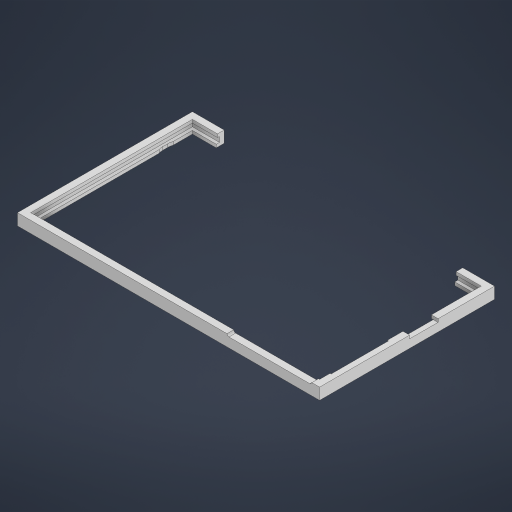
# Autodesk Inventor part: pcb_guard
Saved by Autodesk Inventor 2024 (Build 280153000, 153)
## iProperties
Created: 2024-03-10
Part Number: pcb_guard
Material: Všeobecné
Document SubType Name: Modeling
Designer: Simak
Density: 1 g/cm^3
Appearance: Výchozí
Author: Simak
Autodesk Inventor part; units mm, degrees
ref_plane "YZ Plane" through (0, 0, 0) normal (1, 0, 0) x (0, 1, 0)
ref_plane "XZ Plane" through (0, 0, 0) normal (0, 1, 0) x (-1, 0, 0)
ref_plane "XY Plane" through (0, 0, 0) normal (0, 0, 1) x (1, 0, 0)
sketch "Náčrt1" plane through (0, 0, 0) normal (0, 1, 0) x (-1, 0, 0)
  line L0 (47.5, -27.5) -> (-47.5, -27.5) construction
  line L1 (-47.5, -27.5) -> (-47.5, 27.5) construction
  line L2 (-47.5, 27.5) -> (47.5, 27.5) construction
  line L3 (47.5, 27.5) -> (47.5, -27.5) construction
  line L4 (47.5, -27.5) -> (0, 0) construction
  line L5 (0, 0) -> (-47.5, -27.5) construction
  line L6 (0, 0) -> (-47.5, 27.5) construction
  line L7 (-46, -26) -> (46, -26)
  line L8 (46, -26) -> (46, 26)
  line L9 (46, 26) -> (-46, 26)
  line L10 (-46, 26) -> (-46, -26)
  circle A0 centre (41, -16) radius 4.25
  circle A1 centre (41, -17.5) radius 4.25
  line L11 (45.25, -17.5) -> (45.25, -16)
  line L12 (45, -25) -> (-45, -25)
  line L13 (-45, -25) -> (-45, 25)
  line L14 (-45, 25) -> (45, 25)
  line L15 (45, 25) -> (45, -25)
  line L16 (0, -25) -> (0, 25) construction
  circle A2 centre (-41, -16) radius 4.25
  circle A3 centre (-41, -17.5) radius 4.25
  line L17 (-45.25, -17.5) -> (-45.25, -16)
  line L18 (47.5, -27.5) -> (-47.5, -27.5)
  line L19 (-47.5, -27.5) -> (-47.5, 27.5)
  line L20 (-47.5, 27.5) -> (47.5, 27.5)
  line L21 (47.5, 27.5) -> (47.5, -27.5)
  line L22 (37.5, -27.5) -> (37.5, -25)
  line L23 (-37.5, -25) -> (-37.5, -27.5)
  point P0 (45, -18.9361)
  point P1 (-45, -18.9361)
  point P2 (-45, -14.5639)
  point P3 (45, -14.5639)
  point P4 (-37.5, -26)
  point P5 (37.5, -26)
  dimension "d7" = 8.5
  dimension "d0" = 95
  dimension "d1" = 55
  dimension "d2" = 1.5
  dimension "d5" = 10
  dimension "d6" = 17.5
  dimension "d8" = 5
  dimension "d9" = 1
  dimension "d10" = 1.5
  dimension "d15" = 10
  dimension "d16" = 10
  constraints: 48 end point, 8 parallel, 6 perpendicular, 5 point on line, 4 symmetric about line, 4 vertical, 2 equal length, 2 midpoint, 1 horizontal, 1 vertical alignment, 21 other
  measures "d0" distance of L0.start L0.end
  measures "d1" distance of L0.end L1.end
  measures "d2" distance between parallel lines of L0 L7
  measures "d5" distance from line of L7 point (41, -16)
  measures "d6" vertical distance of L4.end point (41, -17.5)
  measures "d8" distance from line of point (41, -17.5) L8
  measures "d9" distance between parallel lines of L7 L12
  measures "d10" distance between parallel lines of L7 L18
  measures "d15" distance between parallel lines of L21 L22
  measures "d16" distance between parallel lines of L19 L23
extrude "Vysunutí1" add sketch "Náčrt1" along normal blind 1 contours L10 L9 L8 L7 L22 L12 L15 A1 L11 A0 L14 L13 A2 L17 A3 L23
extrude "Vysunutí2" add sketch "Náčrt1" along normal blind 2.6 contours L7 L23 L18 L19 L20 L21 L22 L8 L9 L10
sketch "Náčrt2" plane through (0, 2.6, 0) normal (0, 1, 0) x (1, 0, 0)
  line L0 (46, -26) -> (-46, -26) projected
  line L1 (-46, -26) -> (-46, 26) projected
  line L2 (-46, 26) -> (-37.5, 26) projected
  line L3 (-37.5, 26) -> (-37.5, 27.5) projected
  line L4 (-37.5, 27.5) -> (-47.5, 27.5) projected
  line L5 (-47.5, 27.5) -> (-47.5, -27.5) projected
  line L6 (-47.5, -27.5) -> (47.5, -27.5) projected
  line L7 (47.5, -27.5) -> (47.5, 27.5) projected
  line L8 (47.5, 27.5) -> (37.5, 27.5) projected
  line L9 (37.5, 27.5) -> (37.5, 26) projected
  line L10 (37.5, 26) -> (46, 26) projected
  line L11 (46, 26) -> (46, -26) projected
  line L12 (20.25, -4.1) -> (45.75, -4.1)
  line L13 (45.75, -4.1) -> (45.75, -22.1)
  line L14 (45.75, -22.1) -> (20.25, -22.1)
  line L15 (20.25, -22.1) -> (20.25, -4.1)
  line L16 (39.45, -22.5) -> (43.45, -22.5)
  line L17 (43.45, -22.5) -> (43.45, -25)
  line L18 (43.45, -25) -> (39.45, -25)
  line L19 (39.45, -25) -> (39.45, -22.5)
  line L20 (29.7, -22.5) -> (33.7, -22.5)
  line L21 (33.7, -22.5) -> (33.7, -25)
  line L22 (33.7, -25) -> (29.7, -25)
  line L23 (29.7, -25) -> (29.7, -22.5)
  line L24 (20, -22.5) -> (24, -22.5)
  line L25 (24, -22.5) -> (24, -25)
  line L26 (24, -25) -> (20, -25)
  line L27 (20, -25) -> (20, -22.5)
  line L28 (38.615, 9.745) -> (46.52, 9.745)
  line L29 (46.52, 9.745) -> (46.52, 0.805)
  line L30 (46.52, 0.805) -> (38.615, 0.805)
  line L31 (38.615, 0.805) -> (38.615, 9.745)
  line L32 (45.4, 25.4) -> (36.9, 25.4)
  line L33 (36.9, 25.4) -> (36.9, 28.1)
  line L34 (36.9, 28.1) -> (48.1, 28.1)
  line L35 (48.1, 28.1) -> (48.1, -28.1)
  line L36 (48.1, -28.1) -> (-48.1, -28.1)
  line L37 (-48.1, -28.1) -> (-48.1, 28.1)
  line L38 (-48.1, 28.1) -> (-36.9, 28.1)
  line L39 (-36.9, 28.1) -> (-36.9, 25.4)
  line L40 (-36.9, 25.4) -> (-45.4, 25.4)
  line L41 (-45.4, 25.4) -> (-45.4, -25.4)
  line L42 (-45.4, -25.4) -> (45.4, -25.4)
  line L43 (45.4, -25.4) -> (45.4, 25.4)
  line L44 (46, 26) -> (37.5, 26) projected
  line L45 (37.5, 26) -> (37.5, 25) projected
  line L46 (37.5, 25) -> (45, 25) projected
  line L47 (45, 25) -> (45, 18.9361) projected
  arc A0 (45.25, 17.5) -> (45, 18.9361) centre (41, 17.5) ccw projected
  line L48 (45.25, 17.5) -> (45.25, 16) projected
  arc A1 (45, 14.5639) -> (45.25, 16) centre (41, 16) ccw projected
  line L49 (45, 14.5639) -> (45, -25) projected
  line L50 (45, -25) -> (-45, -25) projected
  line L51 (-45, -25) -> (-45, 14.5639) projected
  arc A2 (-45.25, 16) -> (-45, 14.5639) centre (-41, 16) ccw projected
  line L52 (-45.25, 16) -> (-45.25, 17.5) projected
  arc A3 (-45, 18.9361) -> (-45.25, 17.5) centre (-41, 17.5) ccw projected
  line L53 (-45, 18.9361) -> (-45, 25) projected
  line L54 (-45, 25) -> (-37.5, 25) projected
  line L55 (-37.5, 25) -> (-37.5, 26) projected
  line L56 (-37.5, 26) -> (-46, 26) projected
  line L57 (-46, 26) -> (-46, -26) projected
  line L58 (-46, -26) -> (46, -26) projected
  line L59 (46, -26) -> (46, 26) projected
  line L60 (46.52, 9.745) -> (48.1, 9.745)
  line L61 (46.52, 0.805) -> (48.1, 0.805)
  point P0 (0, 0)
  point P1 (43.45, -23.75)
  point P2 (37.5, 25.4)
  point P3 (45.4, 9.745)
  point P4 (45.4, 0.805)
  point P5 (45.4, -4.1)
  point P6 (45.4, -22.1)
  point P7 (-37.5, 25.4)
  point P8 (47.5, 0.805)
  point P9 (47.5, 9.745)
  dimension "d17" = 25.5
  dimension "d19" = 3.9
  dimension "d20" = 30.1
  dimension "d21" = 0.25
  dimension "d22" = 2.5
  dimension "d23" = 2.5
  dimension "d24" = 2.5
  dimension "d25" = 2.55
  dimension "d26" = 4
  dimension "d27" = 1
  dimension "d28" = 5.75
  dimension "d29" = 5.7
  dimension "d30" = 4
  dimension "d31" = 4
  dimension "d33" = 16.255
  dimension "d34" = 26.805
  dimension "d35" = 0.52
  dimension "d36" = 7.905
  dimension "d37" = 0.6
  constraints: 68 end point, 10 parallel, 7 perpendicular, 5 horizontal, 3 point on line, 1 horizontal alignment, 1 midpoint, 11 other
  measures "d17" distance of L13.end L14.end
  measures "d19" distance between parallel lines of L0 L14
  measures "d20" distance between parallel lines of L12 L10
  measures "d21" distance between parallel lines of L11 L13
  measures "d22" distance of L18.end L16.start
  measures "d23" distance of L22.end L20.start
  measures "d24" distance of L26.end L24.start
  measures "d25" distance from line of L11 point (43.45, -23.75)
  measures "d26" distance of L17.end L18.end
  measures "d27" distance between parallel lines of L0 L18
  measures "d28" distance between parallel lines of L19 L21
  measures "d29" distance between parallel lines of L25 L23
  measures "d30" distance of L21.end L22.end
  measures "d31" distance of L25.end L26.end
  measures "d33" distance between parallel lines of L10 L28
  measures "d34" distance between parallel lines of L30 L0
  measures "d35" distance between parallel lines of L11 L29
  measures "d36" distance of L28.start L28.end
  measures "d37" distance between parallel lines of L10 L32
extrude "Vysunutí3" add sketch "Náčrt2" along normal blind 1 contours L11 L30 L61 L7 L6 L5 L4 L3 L2 L1 L0 | L0 L1 L2 L55 L40 L41 L42 L43 L14 L13 L12 L30 L11 | L28 L43 L32 L45 L10 L11 | L11 L10 L9 L8 L7 L60 L28
sketch "Náčrt3" plane through (-47.5, 0, 27.5) normal (0, 0, 1) x (1, 0, 0)
  line L0 (66.5, 3) -> (91.95, 3)
  line L1 (92.9, 3.6) -> (2.1, 3.6) projected
  arc A0 (65.9, 3.6) -> (66.5, 3) centre (66.5, 3.6) ccw
  arc A1 (91.95, 3) -> (92.55, 3.6) centre (91.95, 3.6) ccw
  line L2 (66.5, 3.6) -> (67.5, 2.6) construction
  line L3 (91.95, 3.6) -> (90.95, 2.6) construction
  point P0 (47.5, 0)
  point P1 (67.5, 2.6)
  point P2 (90.95, 2.6)
  dimension "d40" = 0.6
  dimension "d41" = 1
  constraints: 6 end point, 4 point on circle, 4 point on line, 2 centre point, 2 vertical alignment, 1 horizontal, 1 perpendicular
  measures "d40" distance between parallel lines of L1 L0
  measures "d41" horizontal distance of L0.start point (67.5, 2.6)
extrude "Vysunutí4" cut sketch "Náčrt3" against normal up to next
equation "\"d23\" = d22"
equation "\"d24\" = d22"
equation "\"d30\" = d26"
equation "\"d31\" = d26"
